Autodesk Inventor part; units mm, degrees
(part 3 of 3)
  line L457 (12.6921, 17.012) -> (12.6575, 16.8083)
  line L458 (12.6575, 16.8083) -> (12.605, 16.5408)
  line L459 (12.605, 16.5408) -> (12.545, 16.278)
  line L460 (12.545, 16.278) -> (12.4775, 16.0205)
  line L461 (12.4775, 16.0205) -> (12.402, 15.7684)
  line L462 (12.402, 15.7684) -> (12.3182, 15.5224)
  line L463 (12.3182, 15.5224) -> (12.2255, 15.2831)
  line L464 (12.2255, 15.2831) -> (12.123, 15.0512)
  line L465 (12.123, 15.0512) -> (12.0675, 14.9386)
  line L466 (12.0675, 14.9386) -> (12.0089, 14.8285)
  line L467 (12.0089, 14.8285) -> (11.9465, 14.7213)
  line L468 (11.9465, 14.7213) -> (11.9136, 14.6692)
  line L469 (11.9136, 14.6692) -> (11.8792, 14.6183)
  line L470 (11.8792, 14.6183) -> (12.0586, 14.3908)
  line L471 (12.0586, 14.3908) -> (12.3272, 14.1614)
  line L472 (12.3272, 14.1614) -> (12.58, 14.0197)
  line L473 (12.58, 14.0197) -> (12.6249, 14.0617)
  line L474 (12.6249, 14.0617) -> (12.6712, 14.1024)
  line L475 (12.6712, 14.1024) -> (12.7673, 14.1807)
  line L476 (12.7673, 14.1807) -> (12.8669, 14.2559)
  line L477 (12.8669, 14.2559) -> (12.9695, 14.3282)
  line L478 (12.9695, 14.3282) -> (13.1824, 14.4658)
  line L479 (13.1824, 14.4658) -> (13.4043, 14.5948)
  line L480 (13.4043, 14.5948) -> (13.6342, 14.7161)
  line L481 (13.6342, 14.7161) -> (13.8713, 14.83)
  line L482 (13.8713, 14.83) -> (14.1151, 14.937)
  line L483 (14.1151, 14.937) -> (14.3653, 15.0373)
  line L484 (14.3653, 15.0373) -> (14.6213, 15.131)
  line L485 (14.6213, 15.131) -> (14.8171, 15.1971)
  line L486 (14.8171, 15.1971) -> (15.1971, 14.8171)
  line L487 (15.1971, 14.8171) -> (15.131, 14.6213)
  line L488 (15.131, 14.6213) -> (15.0373, 14.3653)
  line L489 (15.0373, 14.3653) -> (14.937, 14.1151)
  line L490 (14.937, 14.1151) -> (14.83, 13.8713)
  line L491 (14.83, 13.8713) -> (14.7161, 13.6342)
  line L492 (14.7161, 13.6342) -> (14.5948, 13.4043)
  line L493 (14.5948, 13.4043) -> (14.4658, 13.1824)
  line L494 (14.4658, 13.1824) -> (14.3282, 12.9695)
  line L495 (14.3282, 12.9695) -> (14.2559, 12.8669)
  line L496 (14.2559, 12.8669) -> (14.1807, 12.7673)
  line L497 (14.1807, 12.7673) -> (14.1024, 12.6712)
  line L498 (14.1024, 12.6712) -> (14.0617, 12.6249)
  line L499 (14.0617, 12.6249) -> (14.0197, 12.58)
  line L500 (14.0197, 12.58) -> (14.1614, 12.3272)
  line L501 (14.1614, 12.3272) -> (14.3908, 12.0586)
  line L502 (14.3908, 12.0586) -> (14.6183, 11.8792)
  line L503 (14.6183, 11.8792) -> (14.6692, 11.9136)
  line L504 (14.6692, 11.9136) -> (14.7213, 11.9465)
  line L505 (14.7213, 11.9465) -> (14.8285, 12.0089)
  line L506 (14.8285, 12.0089) -> (14.9386, 12.0675)
  line L507 (14.9386, 12.0675) -> (15.0512, 12.123)
  line L508 (15.0512, 12.123) -> (15.283, 12.2255)
  line L509 (15.283, 12.2255) -> (15.5224, 12.3182)
  line L510 (15.5224, 12.3182) -> (15.7684, 12.402)
  line L511 (15.7684, 12.402) -> (16.0205, 12.4775)
  line L512 (16.0205, 12.4775) -> (16.278, 12.545)
  line L513 (16.278, 12.545) -> (16.5408, 12.605)
  line L514 (16.5408, 12.605) -> (16.8083, 12.6575)
  line L515 (16.8083, 12.6575) -> (17.012, 12.6921)
  line L516 (17.012, 12.6921) -> (17.3279, 12.2573)
  line L517 (17.3279, 12.2573) -> (17.232, 12.0743)
  line L518 (17.232, 12.0743) -> (17.0994, 11.836)
  line L519 (17.0994, 11.836) -> (16.9612, 11.6047)
  line L520 (16.9612, 11.6047) -> (16.8174, 11.3806)
  line L521 (16.8174, 11.3806) -> (16.6677, 11.1642)
  line L522 (16.6677, 11.1642) -> (16.512, 10.9562)
  line L523 (16.512, 10.9562) -> (16.3499, 10.7572)
  line L524 (16.3499, 10.7572) -> (16.1807, 10.5684)
  line L525 (16.1807, 10.5684) -> (16.0932, 10.4784)
  line L526 (16.0932, 10.4784) -> (16.0034, 10.3917)
  line L527 (16.0034, 10.3917) -> (15.911, 10.3091)
  line L528 (15.911, 10.3091) -> (15.8635, 10.2697)
  line L529 (15.8635, 10.2697) -> (15.815, 10.2319)
  line L530 (15.815, 10.2319) -> (15.9154, 9.9601)
  line L531 (15.9154, 9.9601) -> (16.1, 9.6589)
  line L532 (16.1, 9.6589) -> (16.2966, 9.4461)
  line L533 (16.2966, 9.4461) -> (16.3523, 9.4722)
  line L534 (16.3523, 9.4722) -> (16.4089, 9.4965)
  line L535 (16.4089, 9.4965) -> (16.5245, 9.5414)
  line L536 (16.5245, 9.5414) -> (16.6424, 9.582)
  line L537 (16.6424, 9.582) -> (16.7624, 9.6192)
  line L538 (16.7624, 9.6192) -> (17.0074, 9.6842)
  line L539 (17.0074, 9.6842) -> (17.2583, 9.7383)
  line L540 (17.2583, 9.7383) -> (17.5144, 9.7826)
  line L541 (17.5144, 9.7826) -> (17.7751, 9.8177)
  line L542 (17.7751, 9.8177) -> (18.0401, 9.8442)
  line L543 (18.0401, 9.8442) -> (18.309, 9.8622)
  line L544 (18.309, 9.8622) -> (18.5814, 9.8722)
  line L545 (18.5814, 9.8722) -> (18.788, 9.8745)
  line L546 (18.788, 9.8745) -> (19.032, 9.3957)
  line L547 (19.032, 9.3957) -> (18.9087, 9.23)
  line L548 (18.9087, 9.23) -> (18.7404, 9.0154)
  line L549 (18.7404, 9.0154) -> (18.5678, 8.8085)
  line L550 (18.5678, 8.8085) -> (18.3907, 8.6097)
  line L551 (18.3907, 8.6097) -> (18.209, 8.4194)
  line L552 (18.209, 8.4194) -> (18.0227, 8.2382)
  line L553 (18.0227, 8.2382) -> (17.8314, 8.067)
  line L554 (17.8314, 8.067) -> (17.6348, 7.907)
  line L555 (17.6348, 7.907) -> (17.5342, 7.8318)
  line L556 (17.5342, 7.8318) -> (17.432, 7.7603)
  line L557 (17.432, 7.7603) -> (17.3278, 7.6932)
  line L558 (17.3278, 7.6932) -> (17.2748, 7.6617)
  line L559 (17.2748, 7.6617) -> (17.221, 7.6319)
  line L560 (17.221, 7.6319) -> (17.2776, 7.3478)
  line L561 (17.2776, 7.3478) -> (17.4127, 7.0214)
  line L562 (17.4127, 7.0214) -> (17.5736, 6.7805)
  line L563 (17.5736, 6.7805) -> (17.6327, 6.7975)
  line L564 (17.6327, 6.7975) -> (17.6925, 6.8127)
  line L565 (17.6925, 6.8127) -> (17.8136, 6.8389)
  line L566 (17.8136, 6.8389) -> (17.9365, 6.8606)
  line L567 (17.9365, 6.8606) -> (18.0608, 6.8785)
  line L568 (18.0608, 6.8785) -> (18.3129, 6.9044)
  line L569 (18.3129, 6.9044) -> (18.5692, 6.9186)
  line L570 (18.5692, 6.9186) -> (18.8291, 6.9223)
  line L571 (18.8291, 6.9223) -> (19.0921, 6.9162)
  line L572 (19.0921, 6.9162) -> (19.3579, 6.9009)
  line L573 (19.3579, 6.9009) -> (19.6263, 6.8767)
  line L574 (19.6263, 6.8767) -> (19.897, 6.8439)
  line L575 (19.897, 6.8439) -> (20.1014, 6.8139)
  line L576 (20.1014, 6.8139) -> (20.2675, 6.3028)
  line L577 (20.2675, 6.3028) -> (20.1198, 6.1583)
  line L578 (20.1198, 6.1583) -> (19.92, 5.9727)
  line L579 (19.92, 5.9727) -> (19.7171, 5.7954)
  line L580 (19.7171, 5.7954) -> (19.5111, 5.6267)
  line L581 (19.5111, 5.6267) -> (19.3019, 5.4672)
  line L582 (19.3019, 5.4672) -> (19.0895, 5.3174)
  line L583 (19.0895, 5.3174) -> (18.8738, 5.1783)
  line L584 (18.8738, 5.1783) -> (18.6546, 5.051)
  line L585 (18.6546, 5.051) -> (18.5435, 4.9925)
  line L586 (18.5435, 4.9925) -> (18.4314, 4.9378)
  line L587 (18.4314, 4.9378) -> (18.3179, 4.8878)
  line L588 (18.3179, 4.8878) -> (18.2606, 4.865)
  line L589 (18.2606, 4.865) -> (18.2028, 4.844)
  line L590 (18.2028, 4.844) -> (18.2143, 4.5545)
  line L591 (18.2143, 4.5545) -> (18.2967, 4.211)
  line L592 (18.2967, 4.211) -> (18.418, 3.9479)
  line L593 (18.418, 3.9479) -> (18.479, 3.9554)
  line L594 (18.479, 3.9554) -> (18.5404, 3.9611)
  line L595 (18.5404, 3.9611) -> (18.6642, 3.968)
  line L596 (18.6642, 3.968) -> (18.7889, 3.9703)
  line L597 (18.7889, 3.9703) -> (18.9145, 3.9685)
  line L598 (18.9145, 3.9685) -> (19.1676, 3.9547)
  line L599 (19.1676, 3.9547) -> (19.4229, 3.9286)
  line L600 (19.4229, 3.9286) -> (19.6802, 3.8916)
  line L601 (19.6802, 3.8916) -> (19.939, 3.8444)
  line L602 (19.939, 3.8444) -> (20.1992, 3.7876)
  line L603 (20.1992, 3.7876) -> (20.4604, 3.7218)
  line L604 (20.4604, 3.7218) -> (20.7227, 3.6471)
  line L605 (20.7227, 3.6471) -> (20.9199, 3.5854)
  line L606 (20.9199, 3.5854) -> (21.0039, 3.0547)
  line L607 (21.0039, 3.0547) -> (20.8355, 2.9351)
  line L608 (20.8355, 2.9351) -> (20.6091, 2.783)
  line L609 (20.6091, 2.783) -> (20.381, 2.6396)
  line L610 (20.381, 2.6396) -> (20.1511, 2.5053)
  line L611 (20.1511, 2.5053) -> (19.9195, 2.3804)
  line L612 (19.9195, 2.3804) -> (19.6863, 2.2657)
  line L613 (19.6863, 2.2657) -> (19.4515, 2.162)
  line L614 (19.4515, 2.162) -> (19.2151, 2.0706)
  line L615 (19.2151, 2.0706) -> (19.0962, 2.0301)
  line L616 (19.0962, 2.0301) -> (18.9769, 1.9937)
  line L617 (18.9769, 1.9937) -> (18.857, 1.9621)
  line L618 (18.857, 1.9621) -> (18.7969, 1.9485)
  line L619 (18.7969, 1.9485) -> (18.7365, 1.9368)
  line L620 (18.7365, 1.9368) -> (18.7025, 1.6491)
  line L621 (18.7025, 1.6491) -> (18.7302, 1.297)
  line L622 (18.7302, 1.297) -> (18.8088, 1.018)
  line L623 (18.8088, 1.018) -> (18.8702, 1.016)
  line L624 (18.8702, 1.016) -> (18.9318, 1.012)
  line L625 (18.9318, 1.012) -> (19.0551, 0.9995)
  line L626 (19.0551, 0.9995) -> (19.1787, 0.9822)
  line L627 (19.1787, 0.9822) -> (19.3024, 0.9608)
  line L628 (19.3024, 0.9608) -> (19.5502, 0.9075)
  line L629 (19.5502, 0.9075) -> (19.7984, 0.8418)
  line L630 (19.7984, 0.8418) -> (20.0467, 0.765)
  line L631 (20.0467, 0.765) -> (20.2949, 0.6779)
  line L632 (20.2949, 0.6779) -> (20.543, 0.5812)
  line L633 (20.543, 0.5812) -> (20.7908, 0.4752)
  line L634 (20.7908, 0.4752) -> (21.0381, 0.3604)
  line L635 (21.0381, 0.3604) -> (21.2232, 0.2687)
  line L636 (21.2232, 0.2687) -> (21.2232, -0.2687)
  line L637 (21.2232, -0.2687) -> (21.0381, -0.3604)
  line L638 (21.0381, -0.3604) -> (20.7908, -0.4752)
  line L639 (20.7908, -0.4752) -> (20.543, -0.5812)
  line L640 (20.543, -0.5812) -> (20.2949, -0.6779)
  line L641 (20.2949, -0.6779) -> (20.0466, -0.765)
  line L642 (20.0466, -0.765) -> (19.7984, -0.8418)
  line L643 (19.7984, -0.8418) -> (19.5502, -0.9075)
  line L644 (19.5502, -0.9075) -> (19.3024, -0.9608)
  line L645 (19.3024, -0.9608) -> (19.1787, -0.9822)
  line L646 (19.1787, -0.9822) -> (19.0551, -0.9995)
  line L647 (19.0551, -0.9995) -> (18.9318, -1.012)
  line L648 (18.9318, -1.012) -> (18.8703, -1.016)
  line L649 (18.8703, -1.016) -> (18.8088, -1.018)
  line L650 (18.8088, -1.018) -> (18.7302, -1.297)
  line L651 (18.7302, -1.297) -> (18.7025, -1.6491)
  line L652 (18.7025, -1.6491) -> (18.7365, -1.9368)
  line L653 (18.7365, -1.9368) -> (18.7969, -1.9485)
  line L654 (18.7969, -1.9485) -> (18.857, -1.9621)
  line L655 (18.857, -1.9621) -> (18.9769, -1.9937)
  line L656 (18.9769, -1.9937) -> (19.0962, -2.0301)
  line L657 (19.0962, -2.0301) -> (19.2151, -2.0706)
  line L658 (19.2151, -2.0706) -> (19.4515, -2.162)
  line L659 (19.4515, -2.162) -> (19.6863, -2.2657)
  line L660 (19.6863, -2.2657) -> (19.9195, -2.3804)
  line L661 (19.9195, -2.3804) -> (20.1511, -2.5053)
  line L662 (20.1511, -2.5053) -> (20.381, -2.6396)
  line L663 (20.381, -2.6396) -> (20.6091, -2.783)
  line L664 (20.6091, -2.783) -> (20.8354, -2.9351)
  line L665 (20.8354, -2.9351) -> (21.0039, -3.0547)
  line L666 (21.0039, -3.0547) -> (20.9199, -3.5854)
  line L667 (20.9199, -3.5854) -> (20.7227, -3.6471)
  line L668 (20.7227, -3.6471) -> (20.4604, -3.7217)
  line L669 (20.4604, -3.7217) -> (20.1992, -3.7876)
  line L670 (20.1992, -3.7876) -> (19.939, -3.8444)
  line L671 (19.939, -3.8444) -> (19.6802, -3.8916)
  line L672 (19.6802, -3.8916) -> (19.4229, -3.9286)
  line L673 (19.4229, -3.9286) -> (19.1676, -3.9547)
  line L674 (19.1676, -3.9547) -> (18.9145, -3.9685)
  line L675 (18.9145, -3.9685) -> (18.7889, -3.9703)
  line L676 (18.7889, -3.9703) -> (18.6642, -3.968)
  line L677 (18.6642, -3.968) -> (18.5404, -3.9611)
  line L678 (18.5404, -3.9611) -> (18.479, -3.9554)
  line L679 (18.479, -3.9554) -> (18.418, -3.9479)
  line L680 (18.418, -3.9479) -> (18.2968, -4.211)
  line L681 (18.2968, -4.211) -> (18.2143, -4.5545)
  line L682 (18.2143, -4.5545) -> (18.2028, -4.844)
  line L683 (18.2028, -4.844) -> (18.2606, -4.865)
  line L684 (18.2606, -4.865) -> (18.3179, -4.8878)
  line L685 (18.3179, -4.8878) -> (18.4313, -4.9378)
  line L686 (18.4313, -4.9378) -> (18.5435, -4.9924)
  line L687 (18.5435, -4.9924) -> (18.6546, -5.051)
  line L688 (18.6546, -5.051) -> (18.8738, -5.1783)
  line L689 (18.8738, -5.1783) -> (19.0895, -5.3174)
  line L690 (19.0895, -5.3174) -> (19.3019, -5.4672)
  line L691 (19.3019, -5.4672) -> (19.5111, -5.6267)
  line L692 (19.5111, -5.6267) -> (19.7171, -5.7954)
  line L693 (19.7171, -5.7954) -> (19.92, -5.9727)
  line L694 (19.92, -5.9727) -> (20.1198, -6.1583)
  line L695 (20.1198, -6.1583) -> (20.2675, -6.3028)
  line L696 (20.2675, -6.3028) -> (20.1014, -6.8139)
  line L697 (20.1014, -6.8139) -> (19.897, -6.8439)
  line L698 (19.897, -6.8439) -> (19.6263, -6.8766)
  line L699 (19.6263, -6.8766) -> (19.3579, -6.9008)
  line L700 (19.3579, -6.9008) -> (19.0921, -6.9162)
  line L701 (19.0921, -6.9162) -> (18.8291, -6.9223)
  line L702 (18.8291, -6.9223) -> (18.5692, -6.9186)
  line L703 (18.5692, -6.9186) -> (18.3129, -6.9044)
  line L704 (18.3129, -6.9044) -> (18.0608, -6.8785)
  line L705 (18.0608, -6.8785) -> (17.9365, -6.8606)
  line L706 (17.9365, -6.8606) -> (17.8136, -6.8389)
  line L707 (17.8136, -6.8389) -> (17.6925, -6.8127)
  line L708 (17.6925, -6.8127) -> (17.6327, -6.7975)
  line L709 (17.6327, -6.7975) -> (17.5736, -6.7805)
  line L710 (17.5736, -6.7805) -> (17.4127, -7.0214)
  line L711 (17.4127, -7.0214) -> (17.2776, -7.3478)
  line L712 (17.2776, -7.3478) -> (17.221, -7.6319)
  line L713 (17.221, -7.6319) -> (17.2748, -7.6617)
  line L714 (17.2748, -7.6617) -> (17.3278, -7.6932)
  line L715 (17.3278, -7.6932) -> (17.432, -7.7603)
  line L716 (17.432, -7.7603) -> (17.5342, -7.8318)
  line L717 (17.5342, -7.8318) -> (17.6348, -7.907)
  line L718 (17.6348, -7.907) -> (17.8314, -8.067)
  line L719 (17.8314, -8.067) -> (18.0227, -8.2382)
  line L720 (18.0227, -8.2382) -> (18.209, -8.4194)
  line L721 (18.209, -8.4194) -> (18.3907, -8.6097)
  line L722 (18.3907, -8.6097) -> (18.5678, -8.8085)
  line L723 (18.5678, -8.8085) -> (18.7404, -9.0154)
  line L724 (18.7404, -9.0154) -> (18.9087, -9.23)
  line L725 (18.9087, -9.23) -> (19.032, -9.3957)
  line L726 (19.032, -9.3957) -> (18.788, -9.8745)
  line L727 (18.788, -9.8745) -> (18.5814, -9.8722)
  line L728 (18.5814, -9.8722) -> (18.309, -9.8622)
  line L729 (18.309, -9.8622) -> (18.0401, -9.8441)
  line L730 (18.0401, -9.8441) -> (17.7751, -9.8177)
  line L731 (17.7751, -9.8177) -> (17.5144, -9.7826)
  line L732 (17.5144, -9.7826) -> (17.2583, -9.7383)
  line L733 (17.2583, -9.7383) -> (17.0074, -9.6842)
  line L734 (17.0074, -9.6842) -> (16.7624, -9.6192)
  line L735 (16.7624, -9.6192) -> (16.6424, -9.582)
  line L736 (16.6424, -9.582) -> (16.5245, -9.5414)
  line L737 (16.5245, -9.5414) -> (16.4089, -9.4965)
  line L738 (16.4089, -9.4965) -> (16.3523, -9.4722)
  line L739 (16.3523, -9.4722) -> (16.2966, -9.4461)
  line L740 (16.2966, -9.4461) -> (16.1, -9.6589)
  line L741 (16.1, -9.6589) -> (15.9154, -9.9601)
  line L742 (15.9154, -9.9601) -> (15.815, -10.2319)
  line L743 (15.815, -10.2319) -> (15.8635, -10.2697)
  line L744 (15.8635, -10.2697) -> (15.911, -10.3091)
  line L745 (15.911, -10.3091) -> (16.0034, -10.3917)
  line L746 (16.0034, -10.3917) -> (16.0932, -10.4784)
  line L747 (16.0932, -10.4784) -> (16.1807, -10.5684)
  line L748 (16.1807, -10.5684) -> (16.3499, -10.7571)
  line L749 (16.3499, -10.7571) -> (16.512, -10.9561)
  line L750 (16.512, -10.9561) -> (16.6677, -11.1642)
  line L751 (16.6677, -11.1642) -> (16.8174, -11.3806)
  line L752 (16.8174, -11.3806) -> (16.9612, -11.6047)
  line L753 (16.9612, -11.6047) -> (17.0994, -11.836)
  line L754 (17.0994, -11.836) -> (17.232, -12.0743)
  line L755 (17.232, -12.0743) -> (17.3279, -12.2573)
  line L756 (17.3279, -12.2573) -> (17.012, -12.6921)
  line L757 (17.012, -12.6921) -> (16.8083, -12.6575)
  line L758 (16.8083, -12.6575) -> (16.5408, -12.605)
  line L759 (16.5408, -12.605) -> (16.278, -12.545)
  line L760 (16.278, -12.545) -> (16.0204, -12.4775)
  line L761 (16.0204, -12.4775) -> (15.7684, -12.402)
  line L762 (15.7684, -12.402) -> (15.5224, -12.3182)
  line L763 (15.5224, -12.3182) -> (15.283, -12.2255)
  line L764 (15.283, -12.2255) -> (15.0512, -12.123)
  line L765 (15.0512, -12.123) -> (14.9386, -12.0675)
  line L766 (14.9386, -12.0675) -> (14.8284, -12.0089)
  line L767 (14.8284, -12.0089) -> (14.7213, -11.9465)
  line L768 (14.7213, -11.9465) -> (14.6692, -11.9136)
  line L769 (14.6692, -11.9136) -> (14.6183, -11.8791)
  line L770 (14.6183, -11.8791) -> (14.3908, -12.0586)
  line L771 (14.3908, -12.0586) -> (14.1614, -12.3272)
  line L772 (14.1614, -12.3272) -> (14.0197, -12.58)
  line L773 (14.0197, -12.58) -> (14.0617, -12.6249)
  line L774 (14.0617, -12.6249) -> (14.1024, -12.6712)
  line L775 (14.1024, -12.6712) -> (14.1807, -12.7673)
  line L776 (14.1807, -12.7673) -> (14.2559, -12.8669)
  line L777 (14.2559, -12.8669) -> (14.3282, -12.9695)
  line L778 (14.3282, -12.9695) -> (14.4658, -13.1824)
  line L779 (14.4658, -13.1824) -> (14.5948, -13.4043)
  line L780 (14.5948, -13.4043) -> (14.7161, -13.6342)
  line L781 (14.7161, -13.6342) -> (14.83, -13.8713)
  line L782 (14.83, -13.8713) -> (14.937, -14.1151)
  line L783 (14.937, -14.1151) -> (15.0373, -14.3653)
  line L784 (15.0373, -14.3653) -> (15.131, -14.6213)
  line L785 (15.131, -14.6213) -> (15.1971, -14.8171)
  line L786 (15.1971, -14.8171) -> (14.8171, -15.1971)
  line L787 (14.8171, -15.1971) -> (14.6213, -15.131)
  line L788 (14.6213, -15.131) -> (14.3653, -15.0373)
  line L789 (14.3653, -15.0373) -> (14.1151, -14.937)
  line L790 (14.1151, -14.937) -> (13.8713, -14.83)
  line L791 (13.8713, -14.83) -> (13.6342, -14.7161)
  line L792 (13.6342, -14.7161) -> (13.4043, -14.5948)
  line L793 (13.4043, -14.5948) -> (13.1824, -14.4658)
  line L794 (13.1824, -14.4658) -> (12.9695, -14.3282)
  line L795 (12.9695, -14.3282) -> (12.8669, -14.2559)
  line L796 (12.8669, -14.2559) -> (12.7673, -14.1807)
  line L797 (12.7673, -14.1807) -> (12.6712, -14.1024)
  line L798 (12.6712, -14.1024) -> (12.6249, -14.0617)
  line L799 (12.6249, -14.0617) -> (12.58, -14.0197)
  line L800 (12.58, -14.0197) -> (12.3272, -14.1614)
  line L801 (12.3272, -14.1614) -> (12.0586, -14.3908)
  line L802 (12.0586, -14.3908) -> (11.8792, -14.6182)
  line L803 (11.8792, -14.6182) -> (11.9136, -14.6692)
  line L804 (11.9136, -14.6692) -> (11.9465, -14.7213)
  line L805 (11.9465, -14.7213) -> (12.0089, -14.8284)
  line L806 (12.0089, -14.8284) -> (12.0675, -14.9386)
  line L807 (12.0675, -14.9386) -> (12.123, -15.0512)
  line L808 (12.123, -15.0512) -> (12.2255, -15.2831)
  line L809 (12.2255, -15.2831) -> (12.3182, -15.5224)
  line L810 (12.3182, -15.5224) -> (12.402, -15.7684)
  line L811 (12.402, -15.7684) -> (12.4775, -16.0205)
  line L812 (12.4775, -16.0205) -> (12.545, -16.278)
  line L813 (12.545, -16.278) -> (12.605, -16.5408)
  line L814 (12.605, -16.5408) -> (12.6575, -16.8083)
  line L815 (12.6575, -16.8083) -> (12.6921, -17.012)
  line L816 (12.6921, -17.012) -> (12.2573, -17.3279)
  line L817 (12.2573, -17.3279) -> (12.0743, -17.232)
  line L818 (12.0743, -17.232) -> (11.836, -17.0994)
  line L819 (11.836, -17.0994) -> (11.6047, -16.9612)
  line L820 (11.6047, -16.9612) -> (11.3806, -16.8174)
  line L821 (11.3806, -16.8174) -> (11.1642, -16.6677)
  line L822 (11.1642, -16.6677) -> (10.9562, -16.512)
  line L823 (10.9562, -16.512) -> (10.7571, -16.3499)
  line L824 (10.7571, -16.3499) -> (10.5684, -16.1807)
  line L825 (10.5684, -16.1807) -> (10.4784, -16.0932)
  line L826 (10.4784, -16.0932) -> (10.3917, -16.0034)
  line L827 (10.3917, -16.0034) -> (10.3091, -15.911)
  line L828 (10.3091, -15.911) -> (10.2697, -15.8635)
  line L829 (10.2697, -15.8635) -> (10.2319, -15.815)
  line L830 (10.2319, -15.815) -> (9.9601, -15.9154)
  line L831 (9.9601, -15.9154) -> (9.6589, -16.1)
  line L832 (9.6589, -16.1) -> (9.4461, -16.2966)
  line L833 (9.4461, -16.2966) -> (9.4722, -16.3523)
  line L834 (9.4722, -16.3523) -> (9.4965, -16.4089)
  line L835 (9.4965, -16.4089) -> (9.5414, -16.5245)
  line L836 (9.5414, -16.5245) -> (9.582, -16.6424)
  line L837 (9.582, -16.6424) -> (9.6192, -16.7624)
  line L838 (9.6192, -16.7624) -> (9.6842, -17.0074)
  line L839 (9.6842, -17.0074) -> (9.7383, -17.2583)
  line L840 (9.7383, -17.2583) -> (9.7826, -17.5144)
  line L841 (9.7826, -17.5144) -> (9.8177, -17.7751)
  line L842 (9.8177, -17.7751) -> (9.8441, -18.0401)
  line L843 (9.8441, -18.0401) -> (9.8622, -18.309)
  line L844 (9.8622, -18.309) -> (9.8722, -18.5814)
  line L845 (9.8722, -18.5814) -> (9.8745, -18.788)
  line L846 (9.8745, -18.788) -> (9.3957, -19.032)
  line L847 (9.3957, -19.032) -> (9.23, -18.9087)
  line L848 (9.23, -18.9087) -> (9.0154, -18.7404)
  line L849 (9.0154, -18.7404) -> (8.8085, -18.5678)
  line L850 (8.8085, -18.5678) -> (8.6097, -18.3907)
  line L851 (8.6097, -18.3907) -> (8.4194, -18.209)
  line L852 (8.4194, -18.209) -> (8.2382, -18.0226)
  line L853 (8.2382, -18.0226) -> (8.067, -17.8314)
  line L854 (8.067, -17.8314) -> (7.907, -17.6348)
  line L855 (7.907, -17.6348) -> (7.8318, -17.5342)
  line L856 (7.8318, -17.5342) -> (7.7603, -17.432)
  line L857 (7.7603, -17.432) -> (7.6932, -17.3278)
  line L858 (7.6932, -17.3278) -> (7.6617, -17.2748)
  line L859 (7.6617, -17.2748) -> (7.6319, -17.2209)
  line L860 (7.6319, -17.2209) -> (7.3478, -17.2776)
  line L861 (7.3478, -17.2776) -> (7.0214, -17.4127)
  line L862 (7.0214, -17.4127) -> (6.7805, -17.5736)
  line L863 (6.7805, -17.5736) -> (6.7975, -17.6327)
  line L864 (6.7975, -17.6327) -> (6.8127, -17.6925)
  line L865 (6.8127, -17.6925) -> (6.8389, -17.8137)
  line L866 (6.8389, -17.8137) -> (6.8606, -17.9365)
  line L867 (6.8606, -17.9365) -> (6.8785, -18.0608)
  line L868 (6.8785, -18.0608) -> (6.9044, -18.3129)
  line L869 (6.9044, -18.3129) -> (6.9186, -18.5692)
  line L870 (6.9186, -18.5692) -> (6.9223, -18.8291)
  line L871 (6.9223, -18.8291) -> (6.9162, -19.0921)
  line L872 (6.9162, -19.0921) -> (6.9009, -19.358)
  line L873 (6.9009, -19.358) -> (6.8767, -19.6263)
  line L874 (6.8767, -19.6263) -> (6.8439, -19.897)
  line L875 (6.8439, -19.897) -> (6.8139, -20.1014)
  line L876 (6.8139, -20.1014) -> (6.3028, -20.2675)
  line L877 (6.3028, -20.2675) -> (6.1583, -20.1198)
  line L878 (6.1583, -20.1198) -> (5.9727, -19.92)
  line L879 (5.9727, -19.92) -> (5.7954, -19.7171)
  line L880 (5.7954, -19.7171) -> (5.6267, -19.5111)
  line L881 (5.6267, -19.5111) -> (5.4672, -19.3019)
  line L882 (5.4672, -19.3019) -> (5.3174, -19.0895)
  line L883 (5.3174, -19.0895) -> (5.1783, -18.8738)
  line L884 (5.1783, -18.8738) -> (5.051, -18.6546)
  line L885 (5.051, -18.6546) -> (4.9924, -18.5435)
  line L886 (4.9924, -18.5435) -> (4.9378, -18.4313)
  line L887 (4.9378, -18.4313) -> (4.8878, -18.3179)
  line L888 (4.8878, -18.3179) -> (4.865, -18.2606)
  line L889 (4.865, -18.2606) -> (4.844, -18.2028)
  line L890 (4.844, -18.2028) -> (4.5545, -18.2143)
  line L891 (4.5545, -18.2143) -> (4.211, -18.2968)
  line L892 (4.211, -18.2968) -> (3.9478, -18.418)
  line L893 (3.9478, -18.418) -> (3.9554, -18.479)
  line L894 (3.9554, -18.479) -> (3.9611, -18.5404)
  line L895 (3.9611, -18.5404) -> (3.968, -18.6642)
  line L896 (3.968, -18.6642) -> (3.9703, -18.7889)
  line L897 (3.9703, -18.7889) -> (3.9685, -18.9145)
  line L898 (3.9685, -18.9145) -> (3.9547, -19.1676)
  line L899 (3.9547, -19.1676) -> (3.9286, -19.4229)
  line L900 (3.9286, -19.4229) -> (3.8916, -19.6802)
  line L901 (3.8916, -19.6802) -> (3.8444, -19.939)
  line L902 (3.8444, -19.939) -> (3.7876, -20.1992)
  line L903 (3.7876, -20.1992) -> (3.7218, -20.4605)
  line L904 (3.7218, -20.4605) -> (3.6471, -20.7227)
  line L905 (3.6471, -20.7227) -> (3.5854, -20.9199)
  line L906 (3.5854, -20.9199) -> (3.0547, -21.0039)
  line L907 (3.0547, -21.0039) -> (2.9351, -20.8354)
  line L908 (2.9351, -20.8354) -> (2.783, -20.6091)
  line L909 (2.783, -20.6091) -> (2.6396, -20.381)
  line L910 (2.6396, -20.381) -> (2.5053, -20.1511)
  line L911 (2.5053, -20.1511) -> (2.3804, -19.9195)
  line L912 (2.3804, -19.9195) -> (2.2657, -19.6863)
  line L913 (2.2657, -19.6863) -> (2.162, -19.4515)
  line L914 (2.162, -19.4515) -> (2.0706, -19.2151)
  line L915 (2.0706, -19.2151) -> (2.0301, -19.0962)
  line L916 (2.0301, -19.0962) -> (1.9937, -18.9769)
  line L917 (1.9937, -18.9769) -> (1.9621, -18.857)
  line L918 (1.9621, -18.857) -> (1.9485, -18.7969)
  line L919 (1.9485, -18.7969) -> (1.9368, -18.7365)
  line L920 (1.9368, -18.7365) -> (1.6491, -18.7025)
  line L921 (1.6491, -18.7025) -> (1.2969, -18.7302)
  line L922 (1.2969, -18.7302) -> (1.018, -18.8088)
  line L923 (1.018, -18.8088) -> (1.016, -18.8703)
  line L924 (1.016, -18.8703) -> (1.012, -18.9318)
  line L925 (1.012, -18.9318) -> (0.9995, -19.0551)
  line L926 (0.9995, -19.0551) -> (0.9822, -19.1787)
  line L927 (0.9822, -19.1787) -> (0.9608, -19.3024)
  line L928 (0.9608, -19.3024) -> (0.9075, -19.5502)
  line L929 (0.9075, -19.5502) -> (0.8418, -19.7984)
  line L930 (0.8418, -19.7984) -> (0.765, -20.0467)
  line L931 (0.765, -20.0467) -> (0.6779, -20.2949)
  line L932 (0.6779, -20.2949) -> (0.5812, -20.543)
  line L933 (0.5812, -20.543) -> (0.4752, -20.7908)
  line L934 (0.4752, -20.7908) -> (0.3604, -21.0381)
  line L935 (0.3604, -21.0381) -> (0.2687, -21.2232)
  line L936 (0.2687, -21.2232) -> (-0.2687, -21.2232)
  line L937 (-0.2687, -21.2232) -> (-0.3604, -21.0381)
  line L938 (-0.3604, -21.0381) -> (-0.4752, -20.7908)
  line L939 (-0.4752, -20.7908) -> (-0.5812, -20.543)
  line L940 (-0.5812, -20.543) -> (-0.6779, -20.2949)
  line L941 (-0.6779, -20.2949) -> (-0.765, -20.0467)
  line L942 (-0.765, -20.0467) -> (-0.8418, -19.7984)
  line L943 (-0.8418, -19.7984) -> (-0.9075, -19.5502)
  line L944 (-0.9075, -19.5502) -> (-0.9608, -19.3024)
  line L945 (-0.9608, -19.3024) -> (-0.9822, -19.1787)
  line L946 (-0.9822, -19.1787) -> (-0.9995, -19.0551)
  line L947 (-0.9995, -19.0551) -> (-1.012, -18.9318)
  line L948 (-1.012, -18.9318) -> (-1.016, -18.8702)
  line L949 (-1.016, -18.8702) -> (-1.018, -18.8088)
  line L950 (-1.018, -18.8088) -> (-1.297, -18.7302)
  line L951 (-1.297, -18.7302) -> (-1.6491, -18.7025)
  line L952 (-1.6491, -18.7025) -> (-1.9368, -18.7365)
  line L953 (-1.9368, -18.7365) -> (-1.9485, -18.7969)
  line L954 (-1.9485, -18.7969) -> (-1.9621, -18.857)
  line L955 (-1.9621, -18.857) -> (-1.9937, -18.9769)
  line L956 (-1.9937, -18.9769) -> (-2.0301, -19.0962)
  line L957 (-2.0301, -19.0962) -> (-2.0706, -19.2151)
  line L958 (-2.0706, -19.2151) -> (-2.162, -19.4515)
  line L959 (-2.162, -19.4515) -> (-2.2657, -19.6863)
  line L960 (-2.2657, -19.6863) -> (-2.3804, -19.9195)
  line L961 (-2.3804, -19.9195) -> (-2.5053, -20.1511)
  line L962 (-2.5053, -20.1511) -> (-2.6396, -20.381)
  line L963 (-2.6396, -20.381) -> (-2.783, -20.6091)
  line L964 (-2.783, -20.6091) -> (-2.9351, -20.8354)
  line L965 (-2.9351, -20.8354) -> (-3.0547, -21.0039)
  line L966 (-3.0547, -21.0039) -> (-3.5854, -20.9199)
  line L967 (-3.5854, -20.9199) -> (-3.6471, -20.7227)
  line L968 (-3.6471, -20.7227) -> (-3.7218, -20.4605)
  line L969 (-3.7218, -20.4605) -> (-3.7876, -20.1992)
  line L970 (-3.7876, -20.1992) -> (-3.8444, -19.939)
  line L971 (-3.8444, -19.939) -> (-3.8916, -19.6802)
  line L972 (-3.8916, -19.6802) -> (-3.9286, -19.4229)
  line L973 (-3.9286, -19.4229) -> (-3.9547, -19.1676)
  line L974 (-3.9547, -19.1676) -> (-3.9685, -18.9145)
  line L975 (-3.9685, -18.9145) -> (-3.9703, -18.7889)
  line L976 (-3.9703, -18.7889) -> (-3.968, -18.6642)
  line L977 (-3.968, -18.6642) -> (-3.9611, -18.5404)
  line L978 (-3.9611, -18.5404) -> (-3.9554, -18.479)
  line L979 (-3.9554, -18.479) -> (-3.9479, -18.418)
  line L980 (-3.9479, -18.418) -> (-4.211, -18.2968)
  line L981 (-4.211, -18.2968) -> (-4.5545, -18.2143)
  line L982 (-4.5545, -18.2143) -> (-4.844, -18.2028)
  line L983 (-4.844, -18.2028) -> (-4.865, -18.2606)
  line L984 (-4.865, -18.2606) -> (-4.8878, -18.3179)
  line L985 (-4.8878, -18.3179) -> (-4.9378, -18.4313)
  line L986 (-4.9378, -18.4313) -> (-4.9925, -18.5435)
  line L987 (-4.9925, -18.5435) -> (-5.051, -18.6546)
  line L988 (-5.051, -18.6546) -> (-5.1783, -18.8738)
  line L989 (-5.1783, -18.8738) -> (-5.3174, -19.0895)
  line L990 (-5.3174, -19.0895) -> (-5.4672, -19.3019)
  line L991 (-5.4672, -19.3019) -> (-5.6267, -19.5111)
  line L992 (-5.6267, -19.5111) -> (-5.7954, -19.7171)
  line L993 (-5.7954, -19.7171) -> (-5.9727, -19.92)
  line L994 (-5.9727, -19.92) -> (-6.1584, -20.1198)
  line L995 (-6.1584, -20.1198) -> (-6.3028, -20.2675)
  line L996 (-6.3028, -20.2675) -> (-6.8139, -20.1014)
  line L997 (-6.8139, -20.1014) -> (-6.8439, -19.897)
  line L998 (-6.8439, -19.897) -> (-6.8767, -19.6263)
  line L999 (-6.8767, -19.6263) -> (-6.9009, -19.358)
  line L1000 (-6.9009, -19.358) -> (-6.9162, -19.0921)
  line L1001 (-6.9162, -19.0921) -> (-6.9223, -18.8291)
  line L1002 (-6.9223, -18.8291) -> (-6.9187, -18.5692)
  line L1003 (-6.9187, -18.5692) -> (-6.9044, -18.3129)
  line L1004 (-6.9044, -18.3129) -> (-6.8785, -18.0608)
  line L1005 (-6.8785, -18.0608) -> (-6.8606, -17.9365)
  line L1006 (-6.8606, -17.9365) -> (-6.8389, -17.8137)
  line L1007 (-6.8389, -17.8137) -> (-6.8127, -17.6925)
  line L1008 (-6.8127, -17.6925) -> (-6.7975, -17.6327)
  line L1009 (-6.7975, -17.6327) -> (-6.7805, -17.5736)
  line L1010 (-6.7805, -17.5736) -> (-7.0214, -17.4127)
  line L1011 (-7.0214, -17.4127) -> (-7.3478, -17.2776)
  line L1012 (-7.3478, -17.2776) -> (-7.6319, -17.2209)
  line L1013 (-7.6319, -17.2209) -> (-7.6617, -17.2748)
  line L1014 (-7.6617, -17.2748) -> (-7.6932, -17.3278)
  line L1015 (-7.6932, -17.3278) -> (-7.7603, -17.432)
  line L1016 (-7.7603, -17.432) -> (-7.8318, -17.5342)
  line L1017 (-7.8318, -17.5342) -> (-7.907, -17.6348)
  line L1018 (-7.907, -17.6348) -> (-8.067, -17.8314)
  line L1019 (-8.067, -17.8314) -> (-8.2382, -18.0227)
  line L1020 (-8.2382, -18.0227) -> (-8.4194, -18.209)
  line L1021 (-8.4194, -18.209) -> (-8.6097, -18.3907)
  line L1022 (-8.6097, -18.3907) -> (-8.8085, -18.5678)
  line L1023 (-8.8085, -18.5678) -> (-9.0154, -18.7404)
  line L1024 (-9.0154, -18.7404) -> (-9.23, -18.9087)
  line L1025 (-9.23, -18.9087) -> (-9.3957, -19.032)
  line L1026 (-9.3957, -19.032) -> (-9.8745, -18.788)
  line L1027 (-9.8745, -18.788) -> (-9.8722, -18.5814)
  line L1028 (-9.8722, -18.5814) -> (-9.8622, -18.309)
  line L1029 (-9.8622, -18.309) -> (-9.8441, -18.0401)
  line L1030 (-9.8441, -18.0401) -> (-9.8177, -17.7751)
  line L1031 (-9.8177, -17.7751) -> (-9.7826, -17.5144)
  line L1032 (-9.7826, -17.5144) -> (-9.7383, -17.2583)
  line L1033 (-9.7383, -17.2583) -> (-9.6842, -17.0074)
  line L1034 (-9.6842, -17.0074) -> (-9.6192, -16.7624)
  line L1035 (-9.6192, -16.7624) -> (-9.582, -16.6424)
  line L1036 (-9.582, -16.6424) -> (-9.5414, -16.5245)
  line L1037 (-9.5414, -16.5245) -> (-9.4965, -16.4089)
  line L1038 (-9.4965, -16.4089) -> (-9.4722, -16.3523)
  line L1039 (-9.4722, -16.3523) -> (-9.4461, -16.2966)
  line L1040 (-9.4461, -16.2966) -> (-9.6589, -16.1)
  line L1041 (-9.6589, -16.1) -> (-9.9601, -15.9154)
  line L1042 (-9.9601, -15.9154) -> (-10.2319, -15.815)
  line L1043 (-10.2319, -15.815) -> (-10.2697, -15.8635)
  line L1044 (-10.2697, -15.8635) -> (-10.3091, -15.911)
  line L1045 (-10.3091, -15.911) -> (-10.3917, -16.0034)
  line L1046 (-10.3917, -16.0034) -> (-10.4784, -16.0932)
  line L1047 (-10.4784, -16.0932) -> (-10.5684, -16.1807)
  line L1048 (-10.5684, -16.1807) -> (-10.7572, -16.3499)
  line L1049 (-10.7572, -16.3499) -> (-10.9562, -16.512)
  line L1050 (-10.9562, -16.512) -> (-11.1642, -16.6677)
  line L1051 (-11.1642, -16.6677) -> (-11.3806, -16.8174)
  line L1052 (-11.3806, -16.8174) -> (-11.6047, -16.9612)
  line L1053 (-11.6047, -16.9612) -> (-11.8361, -17.0994)
  line L1054 (-11.8361, -17.0994) -> (-12.0743, -17.232)
  line L1055 (-12.0743, -17.232) -> (-12.2573, -17.3279)
  line L1056 (-12.2573, -17.3279) -> (-12.6921, -17.012)
  line L1057 (-12.6921, -17.012) -> (-12.6575, -16.8083)
  line L1058 (-12.6575, -16.8083) -> (-12.605, -16.5407)
  line L1059 (-12.605, -16.5407) -> (-12.545, -16.278)
  line L1060 (-12.545, -16.278) -> (-12.4775, -16.0205)
  line L1061 (-12.4775, -16.0205) -> (-12.402, -15.7684)
  line L1062 (-12.402, -15.7684) -> (-12.3182, -15.5224)
  line L1063 (-12.3182, -15.5224) -> (-12.2255, -15.2831)
  line L1064 (-12.2255, -15.2831) -> (-12.123, -15.0512)
  line L1065 (-12.123, -15.0512) -> (-12.0675, -14.9386)
  line L1066 (-12.0675, -14.9386) -> (-12.0089, -14.8285)
  line L1067 (-12.0089, -14.8285) -> (-11.9465, -14.7213)
  line L1068 (-11.9465, -14.7213) -> (-11.9136, -14.6692)
  line L1069 (-11.9136, -14.6692) -> (-11.8792, -14.6183)
  line L1070 (-11.8792, -14.6183) -> (-12.0586, -14.3908)
  line L1071 (-12.0586, -14.3908) -> (-12.3272, -14.1614)
  line L1072 (-12.3272, -14.1614) -> (-12.58, -14.0197)
  line L1073 (-12.58, -14.0197) -> (-12.6249, -14.0617)
  line L1074 (-12.6249, -14.0617) -> (-12.6713, -14.1024)
  line L1075 (-12.6713, -14.1024) -> (-12.7673, -14.1807)
  line L1076 (-12.7673, -14.1807) -> (-12.8669, -14.2559)
  line L1077 (-12.8669, -14.2559) -> (-12.9695, -14.3282)
  line L1078 (-12.9695, -14.3282) -> (-13.1824, -14.4658)
  line L1079 (-13.1824, -14.4658) -> (-13.4043, -14.5948)
  line L1080 (-13.4043, -14.5948) -> (-13.6342, -14.7161)
  line L1081 (-13.6342, -14.7161) -> (-13.8713, -14.83)
  line L1082 (-13.8713, -14.83) -> (-14.1151, -14.937)
  line L1083 (-14.1151, -14.937) -> (-14.3653, -15.0373)
  line L1084 (-14.3653, -15.0373) -> (-14.6213, -15.131)
  line L1085 (-14.6213, -15.131) -> (-14.8171, -15.1971)
  line L1086 (-14.8171, -15.1971) -> (-15.1971, -14.8171)
  line L1087 (-15.1971, -14.8171) -> (-15.131, -14.6213)
  line L1088 (-15.131, -14.6213) -> (-15.0373, -14.3653)
  line L1089 (-15.0373, -14.3653) -> (-14.937, -14.1151)
  line L1090 (-14.937, -14.1151) -> (-14.83, -13.8713)
  line L1091 (-14.83, -13.8713) -> (-14.7161, -13.6342)
  line L1092 (-14.7161, -13.6342) -> (-14.5948, -13.4043)
  line L1093 (-14.5948, -13.4043) -> (-14.4658, -13.1824)
  line L1094 (-14.4658, -13.1824) -> (-14.3282, -12.9695)
  line L1095 (-14.3282, -12.9695) -> (-14.2559, -12.8669)
  line L1096 (-14.2559, -12.8669) -> (-14.1807, -12.7673)
  line L1097 (-14.1807, -12.7673) -> (-14.1024, -12.6712)
  line L1098 (-14.1024, -12.6712) -> (-14.0617, -12.6249)
  line L1099 (-14.0617, -12.6249) -> (-14.0197, -12.58)
  line L1100 (-14.0197, -12.58) -> (-14.1614, -12.3272)
  line L1101 (-14.1614, -12.3272) -> (-14.3908, -12.0586)
  line L1102 (-14.3908, -12.0586) -> (-14.6183, -11.8792)
  line L1103 (-14.6183, -11.8792) -> (-14.6692, -11.9136)
  line L1104 (-14.6692, -11.9136) -> (-14.7213, -11.9465)
  line L1105 (-14.7213, -11.9465) -> (-14.8285, -12.0089)
  line L1106 (-14.8285, -12.0089) -> (-14.9386, -12.0675)
  line L1107 (-14.9386, -12.0675) -> (-15.0512, -12.123)
  line L1108 (-15.0512, -12.123) -> (-15.2831, -12.2255)
  line L1109 (-15.2831, -12.2255) -> (-15.5224, -12.3182)
  line L1110 (-15.5224, -12.3182) -> (-15.7684, -12.402)
  line L1111 (-15.7684, -12.402) -> (-16.0205, -12.4775)
  line L1112 (-16.0205, -12.4775) -> (-16.278, -12.545)
  line L1113 (-16.278, -12.545) -> (-16.5408, -12.605)
  line L1114 (-16.5408, -12.605) -> (-16.8083, -12.6575)
  line L1115 (-16.8083, -12.6575) -> (-17.012, -12.6921)
  line L1116 (-17.012, -12.6921) -> (-17.3279, -12.2573)
  line L1117 (-17.3279, -12.2573) -> (-17.232, -12.0743)
  line L1118 (-17.232, -12.0743) -> (-17.0994, -11.836)
  line L1119 (-17.0994, -11.836) -> (-16.9612, -11.6047)
  line L1120 (-16.9612, -11.6047) -> (-16.8174, -11.3806)
  line L1121 (-16.8174, -11.3806) -> (-16.6677, -11.1642)
  line L1122 (-16.6677, -11.1642) -> (-16.512, -10.9561)
  line L1123 (-16.512, -10.9561) -> (-16.3499, -10.7572)
  line L1124 (-16.3499, -10.7572) -> (-16.1807, -10.5684)
  line L1125 (-16.1807, -10.5684) -> (-16.0932, -10.4784)
  line L1126 (-16.0932, -10.4784) -> (-16.0034, -10.3917)
  line L1127 (-16.0034, -10.3917) -> (-15.911, -10.3091)
  line L1128 (-15.911, -10.3091) -> (-15.8635, -10.2697)
  line L1129 (-15.8635, -10.2697) -> (-15.815, -10.2319)
  line L1130 (-15.815, -10.2319) -> (-15.9154, -9.9601)
  line L1131 (-15.9154, -9.9601) -> (-16.1, -9.6589)
  line L1132 (-16.1, -9.6589) -> (-16.2966, -9.4461)
  line L1133 (-16.2966, -9.4461) -> (-16.3523, -9.4722)
  line L1134 (-16.3523, -9.4722) -> (-16.4089, -9.4965)
  line L1135 (-16.4089, -9.4965) -> (-16.5245, -9.5414)
  line L1136 (-16.5245, -9.5414) -> (-16.6424, -9.582)
  line L1137 (-16.6424, -9.582) -> (-16.7624, -9.6192)
  line L1138 (-16.7624, -9.6192) -> (-17.0074, -9.6842)
  line L1139 (-17.0074, -9.6842) -> (-17.2583, -9.7383)
  line L1140 (-17.2583, -9.7383) -> (-17.5144, -9.7826)
  line L1141 (-17.5144, -9.7826) -> (-17.7751, -9.8177)
  line L1142 (-17.7751, -9.8177) -> (-18.0401, -9.8441)
  line L1143 (-18.0401, -9.8441) -> (-18.309, -9.8622)
  line L1144 (-18.309, -9.8622) -> (-18.5814, -9.8722)
  line L1145 (-18.5814, -9.8722) -> (-18.788, -9.8745)
  line L1146 (-18.788, -9.8745) -> (-19.032, -9.3957)
  line L1147 (-19.032, -9.3957) -> (-18.9087, -9.23)
  line L1148 (-18.9087, -9.23) -> (-18.7405, -9.0154)
  line L1149 (-18.7405, -9.0154) -> (-18.5678, -8.8085)
  line L1150 (-18.5678, -8.8085) -> (-18.3907, -8.6097)
  line L1151 (-18.3907, -8.6097) -> (-18.209, -8.4194)
  line L1152 (-18.209, -8.4194) -> (-18.0227, -8.2382)
  line L1153 (-18.0227, -8.2382) -> (-17.8314, -8.067)
  line L1154 (-17.8314, -8.067) -> (-17.6348, -7.907)
  line L1155 (-17.6348, -7.907) -> (-17.5342, -7.8318)
  line L1156 (-17.5342, -7.8318) -> (-17.432, -7.7603)
  line L1157 (-17.432, -7.7603) -> (-17.3278, -7.6932)
  line L1158 (-17.3278, -7.6932) -> (-17.2748, -7.6617)
  line L1159 (-17.2748, -7.6617) -> (-17.221, -7.6319)
  line L1160 (-17.221, -7.6319) -> (-17.2776, -7.3478)
  line L1161 (-17.2776, -7.3478) -> (-17.4127, -7.0214)
  line L1162 (-17.4127, -7.0214) -> (-17.5736, -6.7805)
  line L1163 (-17.5736, -6.7805) -> (-17.6327, -6.7975)
  line L1164 (-17.6327, -6.7975) -> (-17.6925, -6.8127)
  line L1165 (-17.6925, -6.8127) -> (-17.8137, -6.8389)
  line L1166 (-17.8137, -6.8389) -> (-17.9365, -6.8606)
  line L1167 (-17.9365, -6.8606) -> (-18.0608, -6.8785)
  line L1168 (-18.0608, -6.8785) -> (-18.3129, -6.9044)
  line L1169 (-18.3129, -6.9044) -> (-18.5692, -6.9186)
  line L1170 (-18.5692, -6.9186) -> (-18.8291, -6.9223)
  line L1171 (-18.8291, -6.9223) -> (-19.0921, -6.9162)
  line L1172 (-19.0921, -6.9162) -> (-19.358, -6.9009)
  line L1173 (-19.358, -6.9009) -> (-19.6263, -6.8766)
  line L1174 (-19.6263, -6.8766) -> (-19.897, -6.8439)
  line L1175 (-19.897, -6.8439) -> (-20.1014, -6.8139)
  line L1176 (-20.1014, -6.8139) -> (-20.2675, -6.3028)
  line L1177 (-20.2675, -6.3028) -> (-20.1198, -6.1584)
  line L1178 (-20.1198, -6.1584) -> (-19.92, -5.9727)
  line L1179 (-19.92, -5.9727) -> (-19.7171, -5.7954)
  line L1180 (-19.7171, -5.7954) -> (-19.5111, -5.6267)
  line L1181 (-19.5111, -5.6267) -> (-19.3019, -5.4672)
  line L1182 (-19.3019, -5.4672) -> (-19.0895, -5.3174)
  line L1183 (-19.0895, -5.3174) -> (-18.8738, -5.1783)
  line L1184 (-18.8738, -5.1783) -> (-18.6546, -5.051)
  line L1185 (-18.6546, -5.051) -> (-18.5435, -4.9925)
  line L1186 (-18.5435, -4.9925) -> (-18.4314, -4.9378)
  line L1187 (-18.4314, -4.9378) -> (-18.3179, -4.8878)
  line L1188 (-18.3179, -4.8878) -> (-18.2606, -4.865)
  line L1189 (-18.2606, -4.865) -> (-18.2028, -4.844)
  line L1190 (-18.2028, -4.844) -> (-18.2143, -4.5545)
  line L1191 (-18.2143, -4.5545) -> (-18.2968, -4.211)
  line L1192 (-18.2968, -4.211) -> (-18.418, -3.9479)
  line L1193 (-18.418, -3.9479) -> (-18.479, -3.9554)
  line L1194 (-18.479, -3.9554) -> (-18.5404, -3.9611)
  line L1195 (-18.5404, -3.9611) -> (-18.6642, -3.968)
  line L1196 (-18.6642, -3.968) -> (-18.7889, -3.9703)
  line L1197 (-18.7889, -3.9703) -> (-18.9145, -3.9685)
  line L1198 (-18.9145, -3.9685) -> (-19.1676, -3.9547)
  line L1199 (-19.1676, -3.9547) -> (-19.4229, -3.9286)
  line L1200 (-19.4229, -3.9286) -> (-19.6802, -3.8916)
  line L1201 (-19.6802, -3.8916) -> (-19.939, -3.8444)
  line L1202 (-19.939, -3.8444) -> (-20.1992, -3.7876)
  line L1203 (-20.1992, -3.7876) -> (-20.4605, -3.7217)
  line L1204 (-20.4605, -3.7217) -> (-20.7227, -3.6471)
  line L1205 (-20.7227, -3.6471) -> (-20.9199, -3.5854)
  line L1206 (-20.9199, -3.5854) -> (-21.004, -3.0547)
  line L1207 (-21.004, -3.0547) -> (-20.8355, -2.9351)
  line L1208 (-20.8355, -2.9351) -> (-20.6091, -2.783)
  line L1209 (-20.6091, -2.783) -> (-20.381, -2.6396)
  line L1210 (-20.381, -2.6396) -> (-20.1511, -2.5053)
  line L1211 (-20.1511, -2.5053) -> (-19.9195, -2.3804)
  line L1212 (-19.9195, -2.3804) -> (-19.6863, -2.2657)
  line L1213 (-19.6863, -2.2657) -> (-19.4515, -2.162)
  line L1214 (-19.4515, -2.162) -> (-19.2151, -2.0706)
  line L1215 (-19.2151, -2.0706) -> (-19.0962, -2.0301)
  line L1216 (-19.0962, -2.0301) -> (-18.9769, -1.9937)
  line L1217 (-18.9769, -1.9937) -> (-18.857, -1.9621)
  line L1218 (-18.857, -1.9621) -> (-18.7969, -1.9485)
  line L1219 (-18.7969, -1.9485) -> (-18.7365, -1.9368)
  line L1220 (-18.7365, -1.9368) -> (-18.7025, -1.6491)
  line L1221 (-18.7025, -1.6491) -> (-18.7303, -1.297)
  circle A19 centre (0, 0) radius 0.5
  line L1222 (-21.2232, 0) -> (21.2232, 0) construction
  line L1223 (0, -21.2232) -> (0, 21.2232) construction
  dimension "d33" = 1
  dimension "d36" = 360
  constraints: 41 point on circle, 36 end point, 18 centre point, 4 coincident, 4 collinear, 2 concentric, 2 vertical, 1 perpendicular, 76 other
extrude "Extrusion9" add sketch "Sketch10" along normal mid plane 5 contours A0 L16 A4 L17 | L15 A4 L14 A0 | A0 L19 A4 L18 | L12 A4 L13 A0 | A0 L20 A4 L21 | L11 A4 L10 A0 | A0 L3 A2 L2 | L7 A3 L6 A0 | L22 L23 L24 L25 L26 L27 L28 L29 L30 L31 L32 L33 L34 L35 L36 L37 L38 L39 L40 L41 L42 L43 L44 L45 L46 L47 L48 L49 L50 L51 L52 L53 L54 L55 L56 L57 L58 L59 L60 L61 L62 L63 L64 L65 L66 L67 L68 L69 L70 L71 L72 L73 L74 L75 L76 L77 L78 L79 L80 L81 L82 L83 L84 L85 L86 L87 L88 L89 L90 L91 L92 L93 L94 L95 L96 L97 L98 L99 L100 L101 L102 L103 L104 L105 L106 L107 L108 L109 L110 L111 L112 L113 L114 L115 L116 L117 L118 L119 L120 L121 L122 L123 L124 L125 L126 L127 L128 L129 L130 L131 L132 L133 L134 L135 L136 L137 L138 L139 L140 L141 L142 L143 L144 L145 L146 L147 L148 L149 L150 L151 L152 L153 L154 L155 L156 L157 L158 L159 L160 L161 L162 L163 L164 L165 L166 L167 L168 L169 L170 L171 L172 L173 L174 L175 L176 L177 L178 L179 L180 L181 L182 L183 L184 L185 L186 L187 L188 L189 L190 L191 L192 L193 L194 L195 L196 L197 L198 L199 L200 L201 L202 L203 L204 L205 L206 L207 L208 L209 L210 L211 L212 L213 L214 L215 L216 L217 L218 L219 L220 L221 L222 L223 L224 L225 L226 L227 L228 L229 L230 L231 L232 L233 L234 L235 L236 L237 L238 L239 L240 L241 L242 L243 L244 L245 L246 L247 L248 L249 L250 L251 L252 L253 L254 L255 L256 L257 L258 L259 L260 L261 L262 L263 L264 L265 L266 L267 L268 L269 L270 L271 L272 L273 L274 L275 L276 L277 L278 L279 L280 L281 L282 L283 L284 L285 L286 L287 L288 L289 L290 L291 L292 L293 L294 L295 L296 L297 L298 L299 L300 L301 L302 L303 L304 L305 L306 L307 L308 L309 L310 L311 L312 L313 L314 L315 L316 L317 L318 L319 L320 L321 L322 L323 L324 L325 L326 L327 L328 L329 L330 L331 L332 L333 L334 L335 L336 L337 L338 L339 L340 L341 L342 L343 L344 L345 L346 L347 L348 L349 L350 L351 L352 L353 L354 L355 L356 L357 L358 L359 L360 L361 L362 L363 L364 L365 L366 L367 L368 L369 L370 L371 L372 L373 L374 L375 L376 L377 L378 L379 L380 L381 L382 L383 L384 L385 L386 L387 L388 L389 L390 L391 L392 L393 L394 L395 L396 L397 L398 L399 L400 L401 L402 L403 L404 L405 L406 L407 L408 L409 L410 L411 L412 L413 L414 L415 L416 L417 L418 L419 L420 L421 L422 L423 L424 L425 L426 L427 L428 L429 L430 L431 L432 L433 L434 L435 L436 L437 L438 L439 L440 L441 L442 L443 L444 L445 L446 L447 L448 L449 L450 L451 L452 L453 L454 L455 L456 L457 L458 L459 L460 L461 L462 L463 L464 L465 L466 L467 L468 L469 L470 L471 L472 L473 L474 L475 L476 L477 L478 L479 L480 L481 L482 L483 L484 L485 L486 L487 L488 L489 L490 L491 L492 L493 L494 L495 L496 L497 L498 L499 L500 L501 L502 L503 L504 L505 L506 L507 L508 L509 L510 L511 L512 L513 L514 L515 L516 L517 L518 L519 L520 L521 L522 L523 L524 L525 L526 L527 L528 L529 L530 L531 L532 L533 L534 L535 L536 L537 L538 L539 L540 L541 L542 L543 L544 L545 L546 L547 L548 L549 L550 L551 L552 L553 L554 L555 L556 L557 L558 L559 L560 L561 L562 L563 L564 L565 L566 L567 L568 L569 L570 L571 L572 L573 L574 L575 L576 L577 L578 L579 L580 L581 L582 L583 L584 L585 L586 L587 L588 L589 L590 L591 L592 L593 L594 L595 L596 L597 L598 L599 L600 L601 L602 L603 L604 L605 L606 L607 L608 L609 L610 L611 L612 L613 L614 L615 L616 L617 L618 L619 L620 L621 L622 L623 L624 L625 L626 L627 L628 L629 L630 L631 L632 L633 L634 L635 L636 L637 L638 L639 L640 L641 L642 L643 L644 L645 L646 L647 L648 L649 L650 L651 L652 L653 L654 L655 L656 L657 L658 L659 L660 L661 L662 L663 L664 L665 L666 L667 L668 L669 L670 L671 L672 L673 L674 L675 L676 L677 L678 L679 L680 L681 L682 L683 L684 L685 L686 L687 L688 L689 L690 L691 L692 L693 L694 L695 L696 L697 L698 L699 L700 L701 L702 L703 L704 L705 L706 L707 L708 L709 L710 L711 L712 L713 L714 L715 L716 L717 L718 L719 L720 L721 L722 L723 L724 L725 L726 L727 L728 L729 L730 L731 L732 L733 L734 L735 L736 L737 L738 L739 L740 L741 L742 L743 L744 L745 L746 L747 L748 L749 L750 L751 L752 L753 L754 L755 L756 L757 L758 L759 L760 L761 L762 L763 L764 L765 L766 L767 L768 L769 L770 L771 L772 L773 L774 L775 L776 L777 L778 L779 L780 L781 L782 L783 L784 L785 L786 L787 L788 L789 L790 L791 L792 L793 L794 L795 L796 L797 L798 L799 L800 L801 L802 L803 L804 L805 L806 L807 L808 L809 L810 L811 L812 L813 L814 L815 L816 L817 L818 L819 L820 L821 L822 L823 L824 L825 L826 L827 L828 L829 L830 L831 L832 L833 L834 L835 L836 L837 L838 L839 L840 L841 L842 L843 L844 L845 L846 L847 L848 L849 L850 L851 L852 L853 L854 L855 L856 L857 L858 L859 L860 L861 L862 L863 L864 L865 L866 L867 L868 L869 L870 L871 L872 L873 L874 L875 L876 L877 L878 L879 L880 L881 L882 L883 L884 L885 L886 L887 L888 L889 L890 L891 L892 L893 L894 L895 L896 L897 L898 L899 L900 L901 L902 L903 L904 L905 L906 L907 L908 L909 L910 L911 L912 L913 L914 L915 L916 L917 L918 L919 L920 L921 L922 L923 L924 L925 L926 L927 L928 L929 L930 L931 L932 L933 L934 L935 L936 L937 L938 L939 L940 L941 L942 L943 L944 L945 L946 L947 L948 L949 L950 L951 L952 L953 L954 L955 L956 L957 L958 L959 L960 L961 L962 L963 L964 L965 L966 L967 L968 L969 L970 L971 L972 L973 L974 L975 L976 L977 L978 L979 L980 L981 L982 L983 L984 L985 L986 L987 L988 L989 L990 L991 L992 L993 L994 L995 L996 L997 L998 L999 L1000 L1001 L1002 L1003 L1004 L1005 L1006 L1007 L1008 L1009 L1010 L1011 L1012 L1013 L1014 L1015 L1016 L1017 L1018 L1019 L1020 L1021 L1022 L1023 L1024 L1025 L1026 L1027 L1028 L1029 L1030 L1031 L1032 L1033 L1034 L1035 L1036 L1037 L1038 L1039 L1040 L1041 L1042 L1043 L1044 L1045 L1046 L1047 L1048 L1049 L1050 L1051 L1052 L1053 L1054 L1055 L1056 L1057 L1058 L1059 L1060 L1061 L1062 L1063 L1064 L1065 L1066 L1067 L1068 L1069 L1070 L1071 L1072 L1073 L1074 L1075 L1076 L1077 L1078 L1079 L1080 L1081 L1082 L1083 L1084 L1085 L1086 L1087 L1088 L1089 L1090 L1091 L1092 L1093 L1094 L1095 L1096 L1097 L1098 L1099 L1100 L1101 L1102 L1103 L1104 L1105 L1106 L1107 L1108 L1109 L1110 L1111 L1112 L1113 L1114 L1115 L1116 L1117 L1118 L1119 L1120 L1121 L1122 L1123 L1124 L1125 L1126 L1127 L1128 L1129 L1130 L1131 L1132 L1133 L1134 L1135 L1136 L1137 L1138 L1139 L1140 L1141 L1142 L1143 L1144 L1145 L1146 L1147 L1148 L1149 L1150 L1151 L1152 L1153 L1154 L1155 L1156 L1157 L1158 L1159 L1160 L1161 L1162 L1163 L1164 L1165 L1166 L1167 L1168 L1169 L1170 L1171 L1172 L1173 L1174 L1175 L1176 L1177 L1178 L1179 L1180 L1181 L1182 L1183 L1184 L1185 L1186 L1187 L1188 L1189 L1190 L1191 L1192 L1193 L1194 L1195 L1196 L1197 L1198 L1199 L1200 L1201 L1202 L1203 L1204 L1205 L1206 L1207 L1208 L1209 L1210 L1211 L1212 L1213 L1214 L1215 L1216 L1217 L1218 L1219 L1220 L1221
extrude "Extrusion10" add sketch "Sketch10" along normal mid plane 1 contours A0 L17 A4 L15 | A0 L18 A4 L16 | L14 A4 L12 A0 | A0 L21 A4 L19 | L13 A4 L11 A0 | A0 L2 A4 L20 | L10 A4 L7 A0 | A0 L6 A1 L3
body "Solid4"
